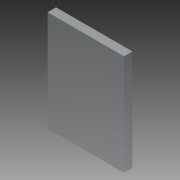
# Autodesk Inventor part: Flight controller
Saved by Autodesk Inventor 2015 (Build 190159000, 159)
## iProperties
Created: 2015-06-20
Part Number: Flight controller
Material: Generic
Document SubType Name: Modeling
Designer: Kristian
Mass: 54.72 g
Surface Area: 163.52 cm^2
Volume: 54.72 cm^3
Density: 1 g/cm^3
Appearance: Clear
Author: Kristian
Autodesk Inventor part; units mm, degrees
ref_plane "YZ Plane" through (0, 0, 0) normal (1, 0, 0) x (0, 1, 0)
ref_plane "XZ Plane" through (0, 0, 0) normal (0, 1, 0) x (-1, 0, 0)
ref_plane "XY Plane" through (0, 0, 0) normal (0, 0, 1) x (1, 0, 0)
sketch "Sketch1" plane through (0, 0, 0) normal (0, 1, 0) x (-1, 0, 0)
  line L0 (-36, 47.5) -> (36, 47.5)
  line L1 (36, 47.5) -> (36, -47.5)
  line L2 (36, -47.5) -> (-36, -47.5)
  line L3 (-36, -47.5) -> (-36, 47.5)
  line L4 (-36, 47.5) -> (36, -47.5) construction
  line L5 (36, 47.5) -> (-36, -47.5) construction
  point P0 (0, 0)
  dimension "d0" = 72
  dimension "d1" = 95
  constraints: 12 end point, 2 midpoint, 2 parallel, 1 horizontal, 1 perpendicular
  measures "d0" distance of L1.end L2.end
  measures "d1" distance of L0.end L1.end
extrude "Extrusion1" add sketch "Sketch1" along normal blind 8
body "Solid1"
